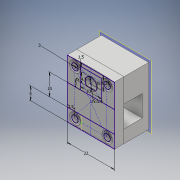
# Autodesk Inventor part: dallas_holder
Saved by Autodesk Inventor 2017 (Build 210142000, 142)
## iProperties
Created: 2020-12-30
Part Number: dallas_holder
Material: Generic
Document SubType Name: Modeling
Designer: arnek
Density: 1 g/cm^3
Appearance: Default
Author: arnek
Autodesk Inventor part; units mm, degrees
ref_plane "YZ Plane" through (0, 0, 0) normal (1, 0, 0) x (0, 1, 0)
ref_plane "XZ Plane" through (0, 0, 0) normal (0, 1, 0) x (-1, 0, 0)
ref_plane "XY Plane" through (0, 0, 0) normal (0, 0, 1) x (1, 0, 0)
sketch "Sketch1" plane through (0, 0, 0) normal (0, 1, 0) x (-1, 0, 0)
  line L0 (0, 0) -> (22, 0)
  line L1 (22, 0) -> (22, -27)
  line L2 (22, -27) -> (0, -27)
  line L3 (0, -27) -> (0, 0)
  arc A0 (13.1213, -8) -> (8.8787, -8) centre (11, -6.25) ccw
  line L4 (13.1213, -8) -> (8.8787, -8)
  line L5 (11, 0) -> (11, -27) construction
  line L6 (0, -21) -> (22, -21)
  line L7 (22, -11) -> (0, -11)
  circle A1 centre (3.5, -24) radius 1.5
  circle A2 centre (18.5, -24) radius 1.5
  circle A3 centre (3.5, -3) radius 1.5
  circle A4 centre (18.5, -3) radius 1.5
  line L8 (3.5, -3) -> (3.5, -24) construction
  line L9 (3.5, -24) -> (18.5, -24) construction
  line L10 (18.5, -24) -> (18.5, -3) construction
  line L11 (18.5, -3) -> (3.5, -3) construction
  line L12 (0, 0) -> (22, -27) construction
  line L13 (18.5, -3) -> (3.5, -24) construction
  line L14 (15.2792, -21) -> (15.2792, -27) construction
  line L15 (16, -1.5) -> (16, -11)
  line L16 (6, -1.5) -> (6, -11)
  line L17 (16, -1.5) -> (6, -11) construction
  line L18 (16, -1.5) -> (6, -1.5)
  point P0 (11, -13.5)
  point P1 (15.2792, -24)
  point P2 (11, -6.25)
  dimension "d1" = 5.5
  dimension "d2" = 4.5
  dimension "d5" = 6.25
  dimension "d6" = 22
  dimension "d8" = 10
  dimension "d9" = 3
  dimension "d10" = 6
  dimension "d11" = 3
  dimension "d12" = 3.5
  dimension "d16" = 10
  dimension "d17" = 1.5
  constraints: 38 end point, 11 point on line, 6 midpoint, 6 perpendicular, 5 centre point, 4 horizontal, 3 equal radius, 3 parallel, 2 point on circle, 2 vertical, 1 coincident
  measures "d1" diameter of A0
  measures "d5" distance from line of L0 A0.centre
  measures "d6" distance of L1.end L2.end
  measures "d8" distance between parallel lines of L6 L7
  measures "d9" distance between parallel lines of L4 L7
  measures "d10" distance between parallel lines of L2 L6
  measures "d11" diameter of A4
  measures "d12" distance from line of L1 L9.end
  measures "d16" distance between parallel lines of L15 L16
  measures "d17" distance between parallel lines of L0 L18
extrude "Extrusion1" add sketch "Sketch1" along normal blind 4.45
sketch "Sketch2" plane through (0, 0, 0) normal (0, 0, 1) x (1, 0, 0)
  arc A0 (0, 0) -> (-22, 0) centre (-11, -149.5961) ccw
  line L0 (0, 0) -> (-22, 0)
  dimension "d20" = 150
  constraints: 2 coincident, 2 end point, 2 point on circle, 1 centre point
  measures "d20" radius of A0
extrude "Extrusion4" cut sketch "Sketch2" against normal through all
ref_plane "Work Plane1" through (0, 15.95, 0) normal (0, 1, 0) x (1, 0, 0)
extrude "Extrusion5" add sketch "Sketch1" along normal up to surface (11.5 mm away) from surface at 4.45 separate body contours L0 L1 L7 L15 L18 L16 L3 | L6 L1 L2 L3
sketch "Sketch3" plane through (0, 15.95, 0) normal (0, 1, 0) x (1, 0, 0)
  line L0 (0, 21) -> (-22, 21) projected
  line L1 (-22, 21) -> (-22, 27) projected
  line L2 (-22, 27) -> (0, 27) projected
  line L3 (0, 27) -> (0, 21) projected
  circle A0 centre (-18.5, 24) radius 1.5 projected
  circle A1 centre (-3.5, 24) radius 1.5 projected
  line L4 (-16, 11) -> (-16, 1.5) projected
  line L5 (-16, 1.5) -> (-6, 1.5) projected
  line L6 (-6, 1.5) -> (-6, 11) projected
  line L7 (-6, 11) -> (0, 11) projected
  line L8 (0, 11) -> (0, 0) projected
  line L9 (0, 0) -> (-22, 0) projected
  line L10 (-22, 0) -> (-22, 11) projected
  line L11 (-22, 11) -> (-16, 11) projected
  circle A2 centre (-3.5, 3) radius 1.5 projected
  circle A3 centre (-18.5, 3) radius 1.5 projected
  line L12 (-6, 11) -> (0, 11) projected
  line L13 (0, 11) -> (0, 21)
  line L14 (0, 0) -> (0, 27) projected
  line L15 (-22, 11) -> (-22, 21)
  constraints: 4 end point, 1 collinear, 1 vertical
extrude "Extrusion6" add sketch "Sketch3" against normal blind 3 contours L13 L7 L6 L5 L4 L11 L15 L0 bodies 2
sketch "Sketch4" plane through (0, 15.95, -27) normal (0, 0, -1) x (-1, 0, 0)
  line L0 (0, -11.5) -> (22, -11.5) projected
  circle A0 centre (11, -11.5) radius 3.5
  point P0 (0, -15.95)
  dimension "d28" = 7
  constraints: 1 centre point, 1 midpoint
  measures "d28" diameter of A0
extrude "Extrusion7" cut sketch "Sketch4" against normal up to surface (6 mm away) bodies 2
sketch "Sketch5" plane through (0, 0, 0) normal (0, 1, 0) x (-1, 0, 0)
  circle A0 centre (3.5, -24) radius 1.5 projected
  circle A1 centre (3.5, -24) radius 2.5
  circle A2 centre (18.5, -24) radius 2.5
  circle A3 centre (18.5, -3) radius 2.5
  circle A4 centre (3.5, -3) radius 1.5 projected
  circle A5 centre (3.5, -3) radius 2.5
  point P0 (0, 0)
  dimension "d31" = 5
  constraints: 4 centre point, 4 coincident, 3 equal radius
  measures "d31" diameter of A1
extrude "Extrusion8" cut sketch "Sketch5" along normal blind 3 bodies 2 1
equation "\"d1\" = dallas_diameter + 2 * Margin"
equation "\"d2\" = dallas_short_diameter + 2 * Margin"
equation "\"Margin\" = 0.5"
equation "\"dallas_diameter\" = 4.5"
equation "\"dallas_short_diameter\" = 3.5"
equation "\"height_part\" = 15.5"
body "Solid1"
body "Solid2"
